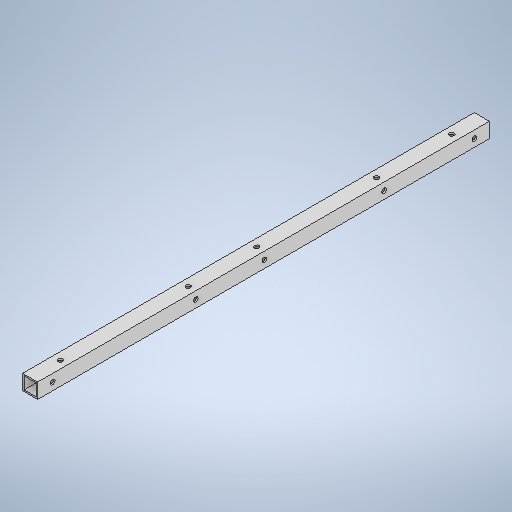
# Autodesk Inventor part: kaku_1010_145
Saved by Autodesk Inventor 2025.1 (Build 291241000, 241)
## iProperties
Created: 2024-11-12
Part Number: kaku_1010_145
Material: 一般
Document SubType Name: Modeling
Designer: yuki0520
Density: 1 g/cm^3
Appearance: 既定
Author: yuki0520
Autodesk Inventor part; units mm, degrees
ref_plane "YZ Plane" through (0, 0, 0) normal (1, 0, 0) x (0, 1, 0)
ref_plane "XZ Plane" through (0, 0, 0) normal (0, 1, 0) x (-1, 0, 0)
ref_plane "XY Plane" through (0, 0, 0) normal (0, 0, 1) x (1, 0, 0)
sketch "スケッチ1" plane through (0, 0, 0) normal (0, 0, 1) x (1, 0, 0)
  line L0 (5, -5) -> (-5, -5)
  line L1 (-5, -5) -> (-5, 5)
  line L2 (-5, 5) -> (5, 5)
  line L3 (5, 5) -> (5, -5)
  line L4 (5, -5) -> (-5, 5) construction
  line L5 (-5, -5) -> (5, 5) construction
  line L6 (4, 4) -> (-4, 4)
  line L7 (-4, 4) -> (-4, -4)
  line L8 (-4, -4) -> (4, -4)
  line L9 (4, -4) -> (4, 4)
  point P0 (0, 0)
  dimension "d0" = 10
  dimension "d1" = 10
  dimension "d2" = 1
  constraints: 20 end point, 4 parallel, 2 midpoint, 2 perpendicular, 1 horizontal, 3 other
  measures "d0" distance of L1.end L2.end
  measures "d1" distance of L0.end L1.end
  measures "d2" distance between parallel lines of L2 L6
extrude "押し出し1" add sketch "スケッチ1" along normal blind 300
sketch "スケッチ2" plane through (5, -5, 0) normal (1, 0, 0) x (0, 0, -1)
  line L0 (0, 5) -> (-300, 5)
  line L1 (0, 1) -> (-300, 1) projected
  line L2 (0, 0) -> (0, 10) projected
  line L3 (-300, 0) -> (-300, 10) projected
  point P0 (-195, 5)
  point P1 (-70, 5)
  point P2 (-150, 5)
  point P3 (-290, 5)
  point P4 (-10, 5)
  point P5 (-149.5, 5)
  dimension "d6" = 125
  dimension "d26" = 80
  dimension "d28" = 10
  dimension "d29" = 10
  dimension "d30" = 280
  dimension "d35" = 79.5
  constraints: 5 point on line, 2 end point, 2 midpoint, 1 parallel
  measures "d6" distance of point (-195, 5) point (-70, 5)
  measures "d26" distance of point (-150, 5) point (-70, 5)
  measures "d28" distance from line of L3 point (-290, 5)
  measures "d29" horizontal distance of L2.end point (-10, 5)
  measures "d30" distance of point (-290, 5) point (-10, 5)
  measures "d35" distance of point (-70, 5) point (-149.5, 5)
hole "穴1" at (5, 0, 195) at (5, 0, 70) at (5, 0, 290) at (5, 0, 10) at (5, 0, 149.5) direction (-1, 0, 0) diameter 3.2 end through all
sketch "スケッチ3" plane through (-5, 5, 0) normal (0, 1, 0) x (1, 0, 0)
  line L0 (5, 0) -> (5, -300)
  line L1 (10, -300) -> (0, -300) projected
  line L2 (10, 0) -> (0, 0) projected
  point P0 (5, -195)
  point P1 (5, -70)
  point P2 (5, -149.5)
  point P3 (5, -150)
  point P4 (5, -20)
  point P5 (5, -280)
  dimension "d15" = 125
  dimension "d27" = 80
  dimension "d31" = 20
  dimension "d32" = 20
  dimension "d33" = 79.5
  dimension "d34" = 50
  constraints: 5 point on line, 2 end point, 2 midpoint
  measures "d15" distance of point (5, -195) point (5, -70)
  measures "d27" distance of point (5, -150) point (5, -70)
  measures "d31" distance from line of L2 point (5, -20)
  measures "d32" distance from line of L1 point (5, -280)
  measures "d33" distance of point (5, -70) point (5, -149.5)
  measures "d34" distance of point (5, -20) point (5, -70)
hole "穴2" at (0, 5, 195) at (0, 5, 70) at (0, 5, 149.5) at (0, 5, 20) at (0, 5, 280) direction (0, -1, 0) diameter 3.2 end through all
equation "\"d32\" = d31"
